Autodesk Inventor part; units mm, degrees
(part 2 of 2)
sketch "Эскиз19" plane through (-553.278877, -264.300199, 1.422232) normal (0, -1, 0) x (1, 0, 0)
  line L0 (41.9631, 0.000002) -> (41.9631, -6.999998)
  line L1 (41.9631, 0.000002) -> (35.9631, 0.000002)
  line L2 (35.9631, -6.999998) -> (35.9631, 0.000002)
  line L3 (41.9631, -6.999998) -> (35.9631, -6.999998)
  circle A0 centre (38.9631, 8.000002) radius 1.75
  line L4 (41.9631, 23.000002) -> (41.9631, 16.000002)
  line L5 (41.9631, 23.000002) -> (35.9631, 23.000002)
  line L6 (35.9631, 16.000002) -> (35.9631, 23.000002)
  line L7 (41.9631, 16.000002) -> (35.9631, 16.000002)
  line L8 (490.372561, 65.867736) -> (-34.635408, 65.867736)
  line L9 (35.9631, 109.000001) -> (35.9631, 116.000001)
  line L10 (41.9631, 109.000001) -> (35.9631, 109.000001)
  line L11 (41.9631, 116.000001) -> (41.9631, 109.000001)
  line L12 (35.9631, 116.000001) -> (41.9631, 116.000001)
  circle A1 centre (38.9631, 124.000001) radius 1.75
  line L13 (41.9631, 132.000001) -> (35.9631, 132.000001)
  line L14 (35.9631, 132.000001) -> (35.9631, 139.000001)
  line L15 (35.9631, 139.000001) -> (41.9631, 139.000001)
  line L16 (41.9631, 139.000001) -> (41.9631, 132.000001)
  line L17 (135.084367, 0.000002) -> (141.084367, 0.000002)
  line L18 (135.084367, -6.999998) -> (135.084367, 0.000002)
  line L19 (135.324736, -6.999997) -> (136.629737, -6.999997)
  line L20 (141.084367, -6.999998) -> (135.084367, -6.999998)
  line L21 (141.084367, 0.000002) -> (141.084367, -6.999998)
  line L22 (135.084367, 16.000002) -> (135.084367, 23.000002)
  line L23 (141.084367, 16.000002) -> (135.084367, 16.000002)
  line L24 (141.084367, 23.000002) -> (141.084367, 16.000002)
  line L25 (135.084367, 23.000002) -> (141.084367, 23.000002)
  circle A2 centre (138.084367, 8.000002) radius 1.75
  line L26 (135.084367, 109.000001) -> (135.084367, 116.000001)
  line L27 (135.084367, 116.000001) -> (141.084367, 116.000001)
  line L28 (141.084367, 109.000001) -> (135.084367, 109.000001)
  line L29 (141.084367, 116.000001) -> (141.084367, 109.000001)
  circle A3 centre (138.383276, 122.178003) radius 0.9
  circle A4 centre (138.084367, 124.000001) radius 1.75
  line L30 (188.226871, 146.409) -> (188.226871, 95.659004)
  line L31 (188.226871, 95.659004) -> (164.226871, 95.659004)
  line L32 (164.226871, 95.659004) -> (164.226871, 146.409)
  line L33 (164.226871, 146.409) -> (188.226871, 146.409)
  line L34 (141.084367, 23.000002) -> (141.084367, 16.000002)
  line L35 (141.084367, 16.000002) -> (135.084367, 16.000002)
  line L36 (135.084367, 16.000002) -> (135.084367, 23.000002)
  line L37 (135.084367, 23.000002) -> (141.084367, 23.000002)
  line L38 (35.9631, 132.000001) -> (35.9631, 139.000001)
  line L39 (35.9631, 139.000001) -> (41.9631, 139.000001)
  line L40 (41.9631, 139.000001) -> (41.9631, 132.000001)
  line L41 (41.9631, 132.000001) -> (35.9631, 132.000001)
  circle A5 centre (38.9631, 8.000002) radius 1.75
  line L42 (41.9631, -6.999998) -> (35.9631, -6.999998)
  line L43 (35.9631, -6.999998) -> (35.9631, 0.000002)
  line L44 (35.9631, 0.000002) -> (41.9631, 0.000002)
  line L45 (41.9631, 0.000002) -> (41.9631, -6.999998)
  line L46 (141.084367, 139.000001) -> (141.084367, 132.000001)
  line L47 (141.084367, 132.000001) -> (135.084367, 132.000001)
  line L48 (135.084367, 132.000001) -> (135.084367, 139.000001)
  line L49 (135.084367, 139.000001) -> (141.084367, 139.000001)
  circle A6 centre (138.084367, 8.000002) radius 1.75
  line L50 (141.084367, 116.000001) -> (141.084367, 109.000001)
  line L51 (141.084367, 109.000001) -> (135.084367, 109.000001)
  line L52 (135.084367, 109.000001) -> (135.084367, 116.000001)
  line L53 (135.084367, 116.000001) -> (141.084367, 116.000001)
  circle A7 centre (38.9631, 124.000001) radius 1.75
  line L54 (41.9631, 16.000002) -> (35.9631, 16.000002)
  line L55 (35.9631, 16.000002) -> (35.9631, 23.000002)
  line L56 (35.9631, 23.000002) -> (41.9631, 23.000002)
  line L57 (41.9631, 23.000002) -> (41.9631, 16.000002)
  line L58 (35.9631, 109.000001) -> (35.9631, 116.000001)
  line L59 (35.9631, 116.000001) -> (41.9631, 116.000001)
  line L60 (41.9631, 116.000001) -> (41.9631, 109.000001)
  line L61 (41.9631, 109.000001) -> (35.9631, 109.000001)
  circle A8 centre (138.084367, 124.000001) radius 1.75
  line L62 (141.084367, 0.000002) -> (141.084367, -6.999998)
  line L63 (141.084367, -6.999998) -> (135.084367, -6.999998)
  line L64 (135.084367, -6.999998) -> (135.084367, 0.000002)
  line L65 (135.084367, 0.000002) -> (141.084367, 0.000002)
  circle A9 centre (130.911055, -16.502322) radius 1.285924
  circle A10 centre (209.546122, 19.017578) radius 1.300502
  circle A11 centre (130.955192, 19.034498) radius 1.251606
  circle A12 centre (209.490361, -16.508496) radius 1.341374
  circle A13 centre (194.523733, 85.500003) radius 1.6
  spline S0 degree 3 poles (38.773733, 66.100003) (38.773733, 66.288728) (38.811522, 66.489786) (38.964711, 66.859248) (39.080092, 67.027682) (39.346051, 67.293641) (39.514486, 67.409025) (39.883953, 67.562215) (40.085014, 67.600003) (40.462453, 67.600003) (40.663513, 67.562215) (41.03298, 67.409025) (41.201416, 67.293641) (41.467375, 67.027682) (41.582756, 66.859248) (41.735944, 66.489786) (41.773733, 66.288728) (41.773733, 65.911278) (41.735944, 65.71022) (41.582756, 65.340758) (41.467375, 65.172324) (41.201416, 64.906365) (41.03298, 64.790982) (40.663513, 64.637791) (40.462453, 64.600003) (40.085014, 64.600003) (39.883953, 64.637791) (39.514486, 64.790982) (39.346051, 64.906365) (39.080092, 65.172324) (38.964711, 65.340758) (38.811522, 65.71022) (38.773733, 65.911278) (38.773733, 66.100003) knots 0 0 0 0 0.05661744 0.05661744 0.11323489 0.11323489 0.16985082 0.16985082 0.22646675 0.22646675 0.28308268 0.28308268 0.33969861 0.33969861 0.39631606 0.39631606 0.4529335 0.4529335 0.50955095 0.50955095 0.56616839 0.56616839 0.62278432 0.62278432 0.67940025 0.67940025 0.73601619 0.73601619 0.79263212 0.79263212 0.84924956 0.84924956 0.905867 0.905867 0.905867 0.905867
  spline S1 degree 3 poles (-19.726267, 65.900003) (-19.726267, 65.711278) (-19.764056, 65.51022) (-19.917244, 65.140758) (-20.032625, 64.972324) (-20.298584, 64.706365) (-20.46702, 64.590982) (-20.836487, 64.437791) (-21.037547, 64.400003) (-21.414986, 64.400003) (-21.616047, 64.437791) (-21.985514, 64.590982) (-22.153949, 64.706365) (-22.419908, 64.972324) (-22.535289, 65.140758) (-22.688478, 65.51022) (-22.726267, 65.711278) (-22.726267, 66.088728) (-22.688478, 66.289786) (-22.535289, 66.659248) (-22.419908, 66.827682) (-22.153949, 67.093641) (-21.985514, 67.209025) (-21.616047, 67.362215) (-21.414986, 67.400003) (-21.037547, 67.400003) (-20.836487, 67.362215) (-20.46702, 67.209025) (-20.298584, 67.093641) (-20.032625, 66.827682) (-19.917244, 66.659248) (-19.764056, 66.289786) (-19.726267, 66.088728) (-19.726267, 65.900003) knots 0 0 0 0 0.05661744 0.05661744 0.11323489 0.11323489 0.16985082 0.16985082 0.22646675 0.22646675 0.28308268 0.28308268 0.33969861 0.33969861 0.39631606 0.39631606 0.4529335 0.4529335 0.50955095 0.50955095 0.56616839 0.56616839 0.62278432 0.62278432 0.67940025 0.67940025 0.73601619 0.73601619 0.79263212 0.79263212 0.84924956 0.84924956 0.905867 0.905867 0.905867 0.905867
  circle A14 centre (132.523733, 149.500003) radius 1.6
  circle A15 centre (132.523733, 37.500003) radius 1.6
  circle A16 centre (132.523733, 85.500003) radius 1.6
  spline S2 degree 3 poles (21.273733, 65.900003) (21.273733, 65.711278) (21.235944, 65.51022) (21.082756, 65.140758) (20.967375, 64.972324) (20.701416, 64.706365) (20.53298, 64.590982) (20.163513, 64.437791) (19.962453, 64.400003) (19.585014, 64.400003) (19.383953, 64.437791) (19.014486, 64.590982) (18.846051, 64.706365) (18.580092, 64.972324) (18.464711, 65.140758) (18.311522, 65.51022) (18.273733, 65.711278) (18.273733, 66.088728) (18.311522, 66.289786) (18.464711, 66.659248) (18.580092, 66.827682) (18.846051, 67.093641) (19.014486, 67.209025) (19.383953, 67.362215) (19.585014, 67.400003) (19.962453, 67.400003) (20.163513, 67.362215) (20.53298, 67.209025) (20.701416, 67.093641) (20.967375, 66.827682) (21.082756, 66.659248) (21.235944, 66.289786) (21.273733, 66.088728) (21.273733, 65.900003) knots 0 0 0 0 0.05661744 0.05661744 0.11323489 0.11323489 0.16985082 0.16985082 0.22646675 0.22646675 0.28308268 0.28308268 0.33969861 0.33969861 0.39631606 0.39631606 0.4529335 0.4529335 0.50955095 0.50955095 0.56616839 0.56616839 0.62278432 0.62278432 0.67940025 0.67940025 0.73601619 0.73601619 0.79263212 0.79263212 0.84924956 0.84924956 0.905867 0.905867 0.905867 0.905867
  spline S3 degree 3 poles (-2.226267, 66.100003) (-2.226267, 66.288728) (-2.188478, 66.489786) (-2.035289, 66.859248) (-1.919908, 67.027682) (-1.653949, 67.293641) (-1.485514, 67.409025) (-1.116047, 67.562215) (-0.914986, 67.600003) (-0.537547, 67.600003) (-0.336487, 67.562215) (0.03298, 67.409025) (0.201416, 67.293641) (0.467375, 67.027682) (0.582756, 66.859248) (0.735944, 66.489786) (0.773733, 66.288728) (0.773733, 65.911278) (0.735944, 65.71022) (0.582756, 65.340758) (0.467375, 65.172324) (0.201416, 64.906365) (0.03298, 64.790982) (-0.336487, 64.637791) (-0.537547, 64.600003) (-0.914986, 64.600003) (-1.116047, 64.637791) (-1.485514, 64.790982) (-1.653949, 64.906365) (-1.919908, 65.172324) (-2.035289, 65.340758) (-2.188478, 65.71022) (-2.226267, 65.911278) (-2.226267, 66.100003) knots 0 0 0 0 0.05661744 0.05661744 0.11323489 0.11323489 0.16985082 0.16985082 0.22646675 0.22646675 0.28308268 0.28308268 0.33969861 0.33969861 0.39631606 0.39631606 0.4529335 0.4529335 0.50955095 0.50955095 0.56616839 0.56616839 0.62278432 0.62278432 0.67940025 0.67940025 0.73601619 0.73601619 0.79263212 0.79263212 0.84924956 0.84924956 0.905867 0.905867 0.905867 0.905867
  circle A17 centre (194.523733, 149.500003) radius 1.6
  circle A18 centre (194.523733, 37.500003) radius 1.6
  line L66 (18.523733, 115.500002) -> (18.523733, 105.500002)
  line L67 (18.523733, 105.500002) -> (-26.476267, 105.500002)
  line L68 (-26.476267, 105.500002) -> (-26.476267, 115.500002)
  line L69 (-26.476267, 115.500002) -> (18.523733, 115.500002)
  line L70 (18.523733, 26.500002) -> (18.523733, 16.500002)
  line L71 (18.523733, 16.500002) -> (-26.476267, 16.500002)
  line L72 (-26.476267, 16.500002) -> (-26.476267, 26.500002)
  line L73 (-26.476267, 26.500002) -> (18.523733, 26.500002)
  circle A19 centre (0, -28.249998) radius 1.75
  circle A20 centre (0, 160.250001) radius 1.75
  circle A21 centre (195.047467, 160.250001) radius 1.75
  circle A22 centre (195.047467, -28.249997) radius 1.75
  circle A23 centre (177.047467, 160.250001) radius 1.75
  circle A24 centre (-18, 160.250001) radius 1.75
  circle A25 centre (-18, -28.249997) radius 1.75
  circle A26 centre (18, 160.250001) radius 1.75
  circle A27 centre (159.047467, -28.249998) radius 1.75
  circle A28 centre (177.047467, -28.249998) radius 1.75
  circle A29 centre (159.047467, 160.250001) radius 1.75
  circle A30 centre (18, -28.249998) radius 1.75
  circle A31 centre (53.523733, 156.000002) radius 5
  circle A32 centre (53.523733, -23.999998) radius 5
  line L74 (66.023733, 157.500002) -> (111.023733, 157.500002)
  line L75 (111.023733, 157.500002) -> (111.023733, -25.499998)
  line L76 (111.023733, -25.499998) -> (66.023733, -25.499998)
  line L77 (66.023733, -25.499998) -> (66.023733, 157.500002)
  line L78 (204.523733, 93.576493) -> (216.523733, 93.576493)
  line L79 (216.523733, 93.576493) -> (216.523733, 38.576493)
  line L80 (216.523733, 38.576493) -> (204.523733, 38.576493)
  line L81 (204.523733, 38.576493) -> (204.523733, 93.576493)
  circle A33 centre (-43.476267, 18.5) radius 1.75
  circle A34 centre (-43.476267, 55.625003) radius 1.75
  circle A35 centre (-43.476267, 113.500003) radius 1.75
  circle A36 centre (-43.476267, 76.375003) radius 1.75
  arc A37 (-38.476267, 163.500003) -> (-46.476267, 155.500003) centre (-38.476267, 155.500003) ccw
  line L82 (-46.476267, 155.500003) -> (-46.476267, 143.500003)
  line L83 (-46.476267, 143.500003) -> (-40.476267, 143.500003)
  line L84 (-40.476267, 143.500003) -> (-40.476267, 123.500003)
  line L85 (-40.476267, 123.500003) -> (-46.476267, 123.500003)
  line L86 (-46.476267, 123.500003) -> (-46.476267, 103.500003)
  line L87 (-46.476267, 103.500003) -> (-40.476267, 103.500003)
  line L88 (-40.476267, 103.500003) -> (-40.476267, 83.500003)
  line L89 (-40.476267, 83.500003) -> (-46.476267, 83.500003)
  line L90 (-46.476267, 83.500003) -> (-46.476267, 48.5)
  line L91 (-46.476267, 48.5) -> (-40.476267, 48.5)
  line L92 (-40.476267, 48.5) -> (-40.476267, 28.5)
  line L93 (-40.476267, 28.5) -> (-46.476267, 28.5)
  line L94 (-46.476267, 28.5) -> (-46.476267, 8.5)
  line L95 (-46.476267, 8.5) -> (-40.476267, 8.5)
  line L96 (-40.476267, 8.5) -> (-40.476267, -11.5)
  line L97 (-40.476267, -11.5) -> (-46.476267, -11.5)
  line L98 (-46.476267, -11.5) -> (-46.476267, -23.499997)
  arc A38 (-46.476267, -23.499997) -> (-38.476267, -31.499997) centre (-38.476267, -23.499997) ccw
  line L99 (-38.476267, -31.499997) -> (26.000003, -31.499999)
  arc A39 (30.000003, -35.5) -> (26.000003, -31.499999) centre (22.7085, -38.791502) ccw
  line L100 (30.000003, -35.5) -> (30.000003, -39)
  arc A40 (30.000003, -39) -> (38.000003, -47) centre (38.000003, -39) ccw
  line L101 (38.000003, -47) -> (138.802962, -47)
  arc A41 (138.802962, -47) -> (146.802962, -39) centre (138.802962, -39) ccw
  line L102 (146.802962, -39) -> (146.802962, -35.499999)
  arc A42 (150.802962, -31.499999) -> (146.802962, -35.499999) centre (154.094465, -38.791502) ccw
  line L103 (150.802962, -31.499999) -> (215.523733, -31.499997)
  arc A43 (215.523733, -31.499997) -> (223.523733, -23.499997) centre (215.523733, -23.499997) ccw
  line L104 (223.523733, -23.499997) -> (223.523733, 155.500003)
  arc A44 (223.523733, 155.500003) -> (215.523733, 163.500003) centre (215.523733, 155.500003) ccw
  line L105 (215.523733, 163.500003) -> (150.802962, 163.500003)
  arc A45 (146.802962, 167.770131) -> (150.802962, 163.500003) centre (154.237087, 170.72543) ccw
  line L106 (146.802962, 167.770131) -> (146.802961, 171.270131)
  arc A46 (146.802961, 171.270131) -> (138.802961, 179.270131) centre (138.802961, 171.270131) ccw
  line L107 (138.802961, 179.270131) -> (38.270127, 179.270131)
  arc A47 (38.270127, 179.270131) -> (30.270127, 171.270131) centre (38.270127, 171.270131) ccw
  line L108 (30.270127, 171.270131) -> (30.270127, 167.770131)
  arc A48 (26, 163.500003) -> (30.270127, 167.770131) centre (22.8966, 170.873531) ccw
  line L109 (26, 163.500003) -> (-38.476267, 163.500003)
  circle A49 centre (111.023733, -35.499998) radius 2
  circle A50 centre (88.523733, -35.499998) radius 2
  circle A51 centre (66.023733, -35.499998) radius 2
  circle A52 centre (111.023733, 167.500002) radius 2
  circle A53 centre (88.523733, 167.500002) radius 2
  circle A54 centre (66.023733, 167.500002) radius 2
  line L110 (130.523733, -6.999999) -> (124.523733, -6.999999)
  line L111 (124.523733, 0.000001) -> (124.523733, -6.999999)
  line L112 (130.523733, 0.000001) -> (124.523733, 0.000001)
  line L113 (130.523733, -6.999999) -> (130.523733, 0.000001)
  line L114 (130.523733, 16.000001) -> (124.523733, 16.000001)
  line L115 (124.523733, 23.000001) -> (124.523733, 16.000001)
  line L116 (130.523733, 23.000001) -> (124.523733, 23.000001)
  line L117 (130.523733, 16.000001) -> (130.523733, 23.000001)
  line L118 (130.523733, 139.000001) -> (124.523733, 139.000001)
  line L119 (130.523733, 132.000001) -> (130.523733, 139.000001)
  line L120 (130.523733, 132.000001) -> (124.523733, 132.000001)
  line L121 (124.523733, 139.000001) -> (124.523733, 132.000001)
  line L122 (130.523733, 116.000001) -> (124.523733, 116.000001)
  line L123 (130.523733, 109.000001) -> (130.523733, 116.000001)
  line L124 (130.523733, 109.000001) -> (124.523733, 109.000001)
  line L125 (124.523733, 116.000001) -> (124.523733, 109.000001)
  line L126 (130.523733, 122.250001) -> (130.523733, 125.750001)
  line L127 (124.523733, 125.750001) -> (124.523733, 122.250001)
  line L128 (130.523733, 6.250001) -> (130.523733, 9.750001)
  line L129 (124.523733, 9.750001) -> (124.523733, 6.250001)
  circle A55 centre (127.523733, 8.000002) radius 1.75
  circle A56 centre (127.523733, 124.000002) radius 1.75
  point P0 (553.278877, -1.422232)
  point P1 (135.336738, -1.986996)
  point P2 (38.773733, 66.100003)
  point P3 (-19.726267, 65.900003)
  point P4 (21.273733, 65.900003)
  point P5 (-2.226267, 66.100003)
  dimension "d23" = 8
  dimension "d24" = 8
  constraints: 40 end point, 12 vertical, 8 horizontal, 2 centre point, 30 other
extrude "Выдавливание18" cut sketch "Эскиз19" against normal blind 8 contours L0 L3 L2 L1 | A0 | L4 L7 L6 L5 | L9 L12 L11 L10 | A1 | L13 L14 L15 L16 | L117 A11 | A11 L117 L114 L115 L116 | L110 L111 L112 L113 | L119 L120 L121 L118 | L123 L124 L125 L122 | A55 | A56 picked at (130.357029, 18.755871)
sketch "Эскиз21" plane through (-553.278877, -260.300199, 1.422232) normal (0, 1, 0) x (1, 0, 0)
  circle A0 centre (20.333024, -160.500002) radius 2
  circle A1 centre (20.333024, -140.500002) radius 2
  circle A2 centre (-3.666976, -160.500002) radius 2
  circle A3 centre (-3.666976, -140.500002) radius 2
  circle A4 centre (20.333024, 8.499998) radius 2
  circle A5 centre (20.333024, 28.499998) radius 2
  circle A6 centre (-3.666976, 8.499998) radius 2
  circle A7 centre (-3.666976, 28.499998) radius 2
  point P0 (553.278877, 1.422232)
extrude "Выдавливание20" cut sketch "Эскиз21" against normal blind 10
chamfer "Фаска2" distance 1 angle 45 4 edges at (-558.9459, -260.3002, -27.0778) (-558.9459, -260.3002, -7.0778) (-534.9459, -260.3002, -27.0778) (-534.9459, -260.3002, -7.0778)
sketch "Эскиз26" plane through (-553.278877, -260.300199, 1.422232) normal (0, 1, 0) x (1, 0, 0)
  line L0 (30.270127, -167.770131) -> (146.802962, -167.770131)
  line L1 (146.802962, -167.770131) -> (30.270127, -167.770131)
  line L2 (30.270127, -167.770131) -> (30.270127, -168.270131)
  line L3 (32.270127, -170.270131) -> (144.802962, -170.270131)
  line L4 (146.802962, -168.270131) -> (146.802962, -167.770131)
  arc A0 (146.802962, 35.5) -> (150.802962, 31.5) centre (154.094465, 38.791502) ccw
  line L5 (146.802962, 35.5) -> (30.000003, 35.5)
  line L6 (30.000003, 35.5) -> (30.000003, 36)
  line L7 (32.000003, 38) -> (144.802962, 38)
  line L8 (146.802962, 36) -> (146.802962, 35.5)
  arc A1 (32.000003, 38) -> (30.000003, 36) centre (32.000003, 36) ccw
  arc A2 (146.802962, 36) -> (144.802962, 38) centre (144.802962, 36) ccw
  arc A3 (144.802962, -170.270131) -> (146.802962, -168.270131) centre (144.802962, -168.270131) ccw
  arc A4 (30.270127, -168.270131) -> (32.270127, -170.270131) centre (32.270127, -168.270131) ccw
  point P0 (553.278877, 1.422232)
  point P1 (50.523733, -167.770131)
  point P2 (146.802962, -170.270131)
  point P3 (30.000003, 38)
  point P4 (50.523733, -167.770131)
  dimension "d91" = 2.5
  dimension "d92" = 2.5
  dimension "d93" = 2
  constraints: 16 end point, 8 point on circle, 8 tangent, 4 centre point, 4 parallel, 4 point on line, 3 equal radius, 2 horizontal, 2 perpendicular
  measures "d91" distance of point (146.803, -170.27) L0.end
  measures "d92" distance of L5.end point (30, 38)
  measures "d93" radius of A1
extrude "Выдавливание25" add sketch "Эскиз26" against normal blind 4
sketch "Эскиз30" plane through (-553.278877, -260.300199, 1.422232) normal (0, 1, 0) x (1, 0, 0)
  line L0 (150.802962, -163.500003) -> (168.523733, -163.500003)
  line L1 (150.802962, -163.500003) -> (19.472488, -163.500003)
  line L2 (19.472488, -163.500003) -> (19.472488, -173.088153)
  line L3 (19.472488, -173.088153) -> (150.802962, -173.088153)
  line L4 (150.802962, -173.088153) -> (150.802962, -163.500003)
  line L5 (168.523733, 31.5) -> (150.802962, 31.5)
  line L6 (150.802962, 31.5) -> (13.110681, 31.5)
  line L7 (13.110681, 31.5) -> (13.110681, 42.898044)
  line L8 (13.110681, 42.898044) -> (150.802962, 42.898044)
  line L9 (150.802962, 42.898044) -> (150.802962, 31.5)
  point P0 (553.278877, 1.422232)
  constraints: 16 end point, 4 parallel, 2 horizontal, 2 perpendicular
sketch "Эскиз32" plane through (-553.278877, -264.300199, 1.422232) normal (0, -1, 0) x (1, 0, 0)
  point P0 (553.278877, -1.422232)
  dimension "d23" = 8
  dimension "d24" = 8
sketch "Эскиз33" plane through (-553.278877, -264.300199, 1.422232) normal (0, -1, 0) x (1, 0, 0)
  arc A0 (150.802962, -31.5) -> (146.802962, -35.5) centre (154.094465, -38.791502) ccw
  line L0 (150.802962, -31.5) -> (26.000003, -31.5)
  line L1 (26.000003, -31.5) -> (26.000003, -41.634712)
  line L2 (26.000003, -41.634712) -> (150.802962, -41.634712)
  line L3 (150.802962, -41.634712) -> (150.802962, -31.5)
  line L4 (-38.476267, 163.500003) -> (26, 163.500003)
  line L5 (26, 163.500003) -> (152.814117, 163.500003)
  line L6 (152.814117, 163.500003) -> (152.814117, 171.954596)
  line L7 (152.814117, 171.954596) -> (26, 171.954596)
  line L8 (26, 171.954596) -> (26, 163.500003)
  point P0 (553.278877, -1.422232)
  dimension "d23" = 8
  dimension "d24" = 8
  constraints: 16 end point, 4 parallel, 2 horizontal, 2 perpendicular
extrude "Выдавливание30" cut sketch "Эскиз33" against normal blind 10
sketch "Эскиз34" plane through (-553.278877, -260.300199, 1.422232) normal (0, 1, 0) x (1, 0, 0)
  line L0 (142.523733, -12.84609) -> (164.523733, -12.84609)
  line L1 (164.523733, -12.84609) -> (164.523733, -18.84609)
  line L2 (164.523733, -18.84609) -> (142.523733, -18.84609)
  line L3 (142.523733, -12.84609) -> (142.523733, -18.84609)
  line L4 (164.523733, -12.84609) -> (142.523733, -12.84609)
  line L5 (142.523733, -12.84609) -> (142.523733, -18.84609)
  line L6 (142.523733, -18.84609) -> (164.523733, -18.84609)
  line L7 (164.523733, -18.84609) -> (164.523733, -12.84609)
  line L8 (176.523733, -155.500003) -> (176.523733, 23.5)
  line L9 (176.523733, 23.5) -> (176.523733, -66)
  line L10 (176.523733, -66) -> (76.13617, -66)
  line L11 (142.523733, -119.153911) -> (164.523733, -119.153911)
  line L12 (164.523733, -119.153911) -> (164.523733, -113.153911)
  line L13 (164.523733, -113.153911) -> (142.523733, -113.153911)
  line L14 (142.523733, -119.153911) -> (142.523733, -113.153911)
  line L15 (164.523733, -119.153911) -> (142.523733, -119.153911)
  line L16 (142.523733, -119.153911) -> (142.523733, -113.153911)
  line L17 (142.523733, -113.153911) -> (164.523733, -113.153911)
  line L18 (164.523733, -113.153911) -> (164.523733, -119.153911)
  point P0 (553.278877, 1.422232)
  dimension "d111" = 89.5
  constraints: 36 end point, 6 symmetric about line, 4 horizontal, 2 parallel, 2 vertical, 1 midpoint, 1 perpendicular, 4 other
  measures "d111" distance of L8.end L9.end
extrude "Выдавливание31" cut sketch "Эскиз34" against normal blind 10
sketch "Эскиз35" plane through (-553.278877, -260.300199, 1.422232) normal (0, 1, 0) x (1, 0, 0)
  line L0 (138.273733, -12.84609) -> (138.273733, -18.84609)
  line L1 (133.273733, -12.84609) -> (133.273733, -18.84609)
  line L2 (139.773733, -12.84609) -> (139.773733, -18.84609)
  line L3 (134.773733, -18.84609) -> (134.773733, -12.84609)
  line L4 (134.773733, -12.84609) -> (138.273733, -12.84609)
  line L5 (138.273733, -12.84609) -> (138.273733, -18.84609)
  line L6 (138.273733, -18.84609) -> (134.773733, -18.84609)
  line L7 (134.773733, -18.84609) -> (134.773733, -12.84609)
  circle A0 centre (136.523733, -15.84609) radius 1.75
  line L8 (142.523733, -12.84609) -> (164.523733, -12.84609)
  line L9 (153.523733, -12.84609) -> (153.523733, -3.062251)
  line L10 (168.773733, -12.84609) -> (168.773733, -18.84609)
  line L11 (173.773733, -12.84609) -> (173.773733, -18.84609)
  line L12 (167.273733, -12.84609) -> (167.273733, -18.84609)
  line L13 (172.273733, -18.84609) -> (172.273733, -12.84609)
  line L14 (172.273733, -12.84609) -> (168.773733, -12.84609)
  line L15 (168.773733, -12.84609) -> (168.773733, -18.84609)
  line L16 (168.773733, -18.84609) -> (172.273733, -18.84609)
  line L17 (172.273733, -18.84609) -> (172.273733, -12.84609)
  circle A1 centre (170.523733, -15.84609) radius 1.75
  line L18 (176.523733, -155.500003) -> (176.523733, 23.5)
  line L19 (176.523733, 23.5) -> (176.523733, -66)
  line L20 (176.523733, -66) -> (84.433717, -66)
  line L21 (138.273733, -119.153911) -> (138.273733, -113.153911)
  line L22 (133.273733, -119.153911) -> (133.273733, -113.153911)
  line L23 (139.773733, -119.153911) -> (139.773733, -113.153911)
  line L24 (134.773733, -113.153911) -> (134.773733, -119.153911)
  line L25 (134.773733, -119.153911) -> (138.273733, -119.153911)
  line L26 (138.273733, -119.153911) -> (138.273733, -113.153911)
  line L27 (138.273733, -113.153911) -> (134.773733, -113.153911)
  line L28 (134.773733, -113.153911) -> (134.773733, -119.153911)
  circle A2 centre (136.523733, -116.153911) radius 1.75
  line L29 (142.523733, -119.153911) -> (164.523733, -119.153911)
  line L30 (153.523733, -119.153911) -> (153.523733, -128.937749)
  line L31 (168.773733, -119.153911) -> (168.773733, -113.153911)
  line L32 (173.773733, -119.153911) -> (173.773733, -113.153911)
  line L33 (167.273733, -119.153911) -> (167.273733, -113.153911)
  line L34 (172.273733, -113.153911) -> (172.273733, -119.153911)
  line L35 (172.273733, -119.153911) -> (168.773733, -119.153911)
  line L36 (168.773733, -119.153911) -> (168.773733, -113.153911)
  line L37 (168.773733, -113.153911) -> (172.273733, -113.153911)
  line L38 (172.273733, -113.153911) -> (172.273733, -119.153911)
  circle A3 centre (170.523733, -116.153911) radius 1.75
  point P0 (553.278877, 1.422232)
  dimension "d112" = 89.5
  constraints: 74 end point, 37 symmetric about line, 5 vertical, 4 centre point, 2 horizontal, 2 midpoint, 2 parallel, 1 perpendicular, 11 other
  measures "d112" distance of L18.end L19.end
extrude "Выдавливание32" cut sketch "Эскиз35" against normal blind 10 contours A0 | A1 | A2 | A3
sketch "Эскиз36" plane through (-553.278877, -260.300199, 1.422232) normal (0, 1, 0) x (1, 0, 0)
  line L0 (166.523733, -81.379789) -> (166.523733, -50.624416)
  line L1 (160.90352, -45.000005) -> (130.148146, -45.000005)
  line L2 (130.143949, -87.000003) -> (160.899322, -87.000003)
  line L3 (124.523735, -50.620219) -> (124.523735, -81.375592)
  line L4 (123.523733, -88.000003) -> (167.523733, -88.000003)
  line L5 (167.523733, -88.000003) -> (167.523733, -44.000003)
  line L6 (167.523733, -44.000003) -> (123.523733, -44.000003)
  line L7 (123.523733, -44.000003) -> (123.523733, -88.000003)
  line L8 (123.523733, -88.000003) -> (167.523733, -44.000003) construction
  line L9 (167.523733, -88.000003) -> (123.523733, -44.000003) construction
  point P0 (553.278877, 1.422232)
  point P1 (145.523733, -66.000003)
  point P2 (145.521636, -87.000003)
  dimension "d115" = 44
  dimension "d116" = 44
  dimension "d117" = 21
  dimension "d118" = 21
  constraints: 20 end point, 3 horizontal, 3 midpoint, 2 parallel, 2 vertical, 1 perpendicular, 8 other
  measures "d115" distance of L5.end L6.end
  measures "d116" distance of L4.end L5.end
  measures "d117" distance from line of L0 point (145.524, -66)
  measures "d118" distance of point (145.522, -87) point (145.524, -66)
extrude "Выдавливание33" cut sketch "Эскиз36" against normal blind 10
